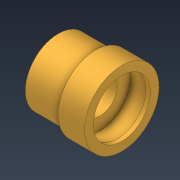
# Autodesk Inventor part: Mocowanie uszczelki przod
Saved by Autodesk Inventor 2022 (Build 260153000, 153)
## iProperties
Created: 2023-04-12
Part Number: Mocowanie uszczelki przod
Material: Brass, Soft Yellow
Document SubType Name: Modeling
Designer: wikto
Density: 8.47 g/cm^3
Appearance: Brass - Satin
Author: wikto
Autodesk Inventor part; units mm, degrees
ref_plane "YZ Plane" through (0, 0, 0) normal (1, 0, 0) x (0, 1, 0)
ref_plane "XZ Plane" through (0, 0, 0) normal (0, 1, 0) x (-1, 0, 0)
ref_plane "XY Plane" through (0, 0, 0) normal (0, 0, 1) x (1, 0, 0)
sketch "Sketch3" plane through (0, 0, 0) normal (0, 0, 1) x (1, 0, 0)
  line L0 (0, 0) -> (100, 0)
  line L1 (0, 8) -> (19, 8)
  line L2 (19, 8) -> (19, 14)
  line L3 (19, 14) -> (27, 14)
  line L4 (27, 14) -> (27, 13)
  line L5 (27, 13) -> (29, 13)
  line L6 (29, 13) -> (29, 17)
  line L7 (29, 17) -> (17, 17)
  line L8 (17, 17) -> (17, 15)
  line L9 (17, 15) -> (0, 15)
  line L10 (0, 15) -> (0, 8)
  dimension "d7" = 100
  dimension "d8" = 29
  dimension "d9" = 2
  dimension "d10" = 8
  dimension "d11" = 12
  dimension "d12" = 3
  dimension "d13" = 4
  dimension "d14" = 7
  dimension "d15" = 16
  dimension "d16" = 28
  constraints: 22 end point, 7 perpendicular, 2 horizontal, 1 parallel, 1 vertical, 1 vertical alignment
  measures "d7" distance of L0.start L0.end
  measures "d8" distance between parallel lines of L10 L6
  measures "d9" distance between parallel lines of L6 L4
  measures "d10" distance between parallel lines of L2 L4
  measures "d11" distance between parallel lines of L8 L6
  measures "d12" distance between parallel lines of L3 L7
  measures "d13" distance between parallel lines of L7 L5
  measures "d14" distance between parallel lines of L9 L1
  measures "d15" diameter of L1 L0
  measures "d16" diameter of L3 L0
revolve "Revolution1" add sketch "Sketch3" angle 360 about axis through (0, 0, 0) along (1, 0, 0)
body "Solid2"
